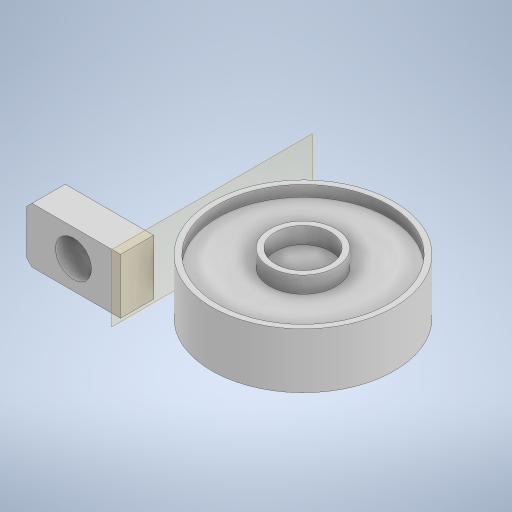
# Autodesk Inventor part: Chumacera con rodamiento 10 mm kp000
Saved by Autodesk Inventor 2024 (Build 280153000, 153)
## iProperties
Created: 2024-04-26
Part Number: Chumacera con rodamiento 10 mm kp000
Material: Genérico
Document SubType Name: Modeling
Designer: alexa
Density: 1 g/cm^3
Appearance: Valor por defecto
Author: alexa
Autodesk Inventor part; units mm, degrees
ref_plane "XZ Plane" through (0, 0, 0) normal (0, 1, 0) x (-1, 0, 0)
ref_plane "XY Plane" through (0, 0, 0) normal (0, 0, 1) x (1, 0, 0)
sketch "Sketch1" plane through (0, 0, 0) normal (0, 1, 0) x (-1, 0, 0)
  circle A0 centre (0, 0) radius 16.5
  dimension "d0" = 33
  constraints: 1 centre point, 1 coincident
  measures "d0" diameter of A0
extrude "Extrusion1" add sketch "Sketch1" along normal blind 8
sketch "Sketch2" plane through (0, 8, 0) normal (0, 1, 0) x (1, 0, 0)
  circle A0 centre (0, 0) radius 16.5
  circle A1 centre (0, 0) radius 15.5
  dimension "d4" = 31
  constraints: 2 centre point, 2 coincident
  measures "d4" diameter of A1
extrude "Extrusion2" add sketch "Sketch2" along normal blind 2
sketch "Sketch3" plane through (0, 8, 0) normal (0, 1, 0) x (1, 0, 0)
  circle A0 centre (0, 0) radius 5
  circle A1 centre (0, 0) radius 6
  dimension "d7" = 10
  dimension "d8" = 12
  constraints: 2 centre point, 2 coincident
  measures "d7" diameter of A0
  measures "d8" diameter of A1
extrude "Extrusion3" add sketch "Sketch3" along normal blind 3
ref_plane "Work Plane1" through (-16.5, 0, 0) normal (1, 0, 0) x (0, 1, 0)
sketch "Sketch4" plane through (-16.5, 0, 0) normal (1, 0, 0) x (0, 1, 0)
  line L0 (0, 16.5) -> (10, 16.5) projected
  line L1 (0, -16.5) -> (0, 16.5) projected
  line L2 (10, 16.5) -> (0, 16.5)
  line L3 (0, 16.5) -> (0, 10.5)
  line L4 (0, 10.5) -> (10, 10.5)
  line L5 (10, 10.5) -> (10, 16.5)
  point P0 (0, 0)
  dimension "d12" = 6
  constraints: 8 end point, 2 parallel, 2 point on line, 1 horizontal, 1 perpendicular
  measures "d12" distance of L3.end L2.end
extrude "Extrusion4" add sketch "Sketch4" against normal blind 17
chamfer "Chamfer1" distance 1 angle 45 2 edges at (-33.5, 10, 13.5) (-33.5, 0, 13.5)
sketch "Sketch5" plane through (-16.5, 0, 10.5) normal (0, 0, -1) x (-1, 0, 0)
  circle A0 centre (8.5, 5.0786) radius 3.25
  point P0 (-16.5, 0)
  dimension "d18" = 6.5
  constraints: 1 centre point
  measures "d18" diameter of A0
extrude "Extrusion5" cut sketch "Sketch5" against normal blind 7
body "Solid1"
